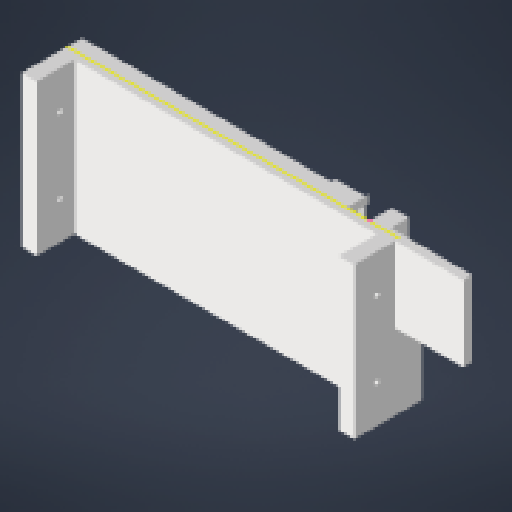
# Autodesk Inventor part: offloadbase
Saved by Autodesk Inventor 2027 (Build 310192000, 192)
## iProperties
Created: 2026-07-10
Part Number: offloadbase
Material: Generic
Document SubType Name: Modeling
Designer: uchiha
Density: 1 g/cm^3
Appearance: Default
Mass: 216.728 g
Surface Area: 672.485 cm^2
Volume: 216.728 cm^3
Author: uchiha
Autodesk Inventor part; units mm, degrees
sketch "Sketch1" plane through (0, 0, 0) normal (0, 0, 1) x (1, 0, 0)
  line L0 (-110, 50) -> (110, 50)
  line L1 (110, 50) -> (110, -50)
  line L2 (110, -50) -> (-110, -50)
  line L3 (-110, -50) -> (-110, 50)
  line L4 (-110, 50) -> (110, -50) construction
  line L5 (110, 50) -> (-110, -50) construction
  line L6 (110, 50) -> (100, 50)
  line L7 (100, 50) -> (100, -50)
  line L8 (100, -50) -> (110, -50)
  line L9 (110, -50) -> (110, 50)
  line L10 (-110, 50) -> (-100, 50)
  line L11 (-100, 50) -> (-100, -50)
  line L12 (-100, -50) -> (-110, -50)
  line L13 (-110, -50) -> (-110, 50)
  point P0 (0, 0)
  dimension "d0" = 220
  dimension "d1" = 100
  dimension "d2" = 10
  dimension "d3" = 10
  constraints: 28 end point, 6 parallel, 3 horizontal, 3 perpendicular, 2 midpoint, 2 point on line
  measures "d0" distance of L1.end L2.end
  measures "d1" distance of L0.end L1.end
  measures "d2" distance of L8.end L7.end
  measures "d3" distance of L11.end L12.end
extrude "Extrusion1" add sketch "Sketch1" along normal blind 5 contours L0 L7 L2 L11
extrude "Extrusion2" add sketch "Sketch1" along normal blind 30 contours L0 L11 L2 L3 | L0 L1 L2 L7
sketch "Sketch2" plane through (110, -50, 0) normal (1, 0, 0) x (0, 0, -1)
  circle A0 centre (-15, 75) radius 1.5
  circle A1 centre (-15, 25) radius 1.5
  line L0 (0, 100) -> (-30, 100) projected
  line L1 (0, 0) -> (-30, 0) projected
  point P0 (0, 50)
  point P1 (-15, 100)
  point P2 (-15, 0)
  dimension "d8" = 3
  dimension "d9" = 3
  dimension "d10" = 25
  dimension "d11" = 25
  constraints: 2 centre point, 2 midpoint
  measures "d8" diameter of A0
  measures "d9" diameter of A1
  measures "d10" distance of point (-15, 100) A0.centre
  measures "d11" distance of point (-15, 0) A1.centre
extrude "Extrusion3" cut sketch "Sketch2" against normal blind 300
ref_plane "Work Plane1" through (0, 0, 2.5) normal (0, 0, -1) x (-1, 0, 0)
sketch "Sketch5" plane through (-100, -50, 5) normal (0, -1, 0) x (1, 0, 0)
  point P0 (100, -5)
sketch "Sketch6" plane through (0, 0, 0) normal (0, 0, -1) x (-1, 0, 0)
  line L0 (-110, 50) -> (110, 50) projected
  line L1 (-90, 50) -> (-75, 50)
  point P0 (0, 0)
  constraints: 2 end point, 1 horizontal
sketch "Sketch7" plane through (-100, -50, 5) normal (0, -1, 0) x (1, 0, 0)
  point P0 (100, -5)
sketch "Sketch10" plane through (0, 0, 0) normal (0, 0, -1) x (-1, 0, 0)
  point P0 (0, 0)
sketch "Sketch11" plane through (-100, -50, 5) normal (0, -1, 0) x (1, 0, 0)
  point P0 (100, -5)
sketch "Sketch12" plane through (-100, -50, 5) normal (0, -1, 0) x (1, 0, 0)
  point P0 (100, -5)
sketch "Sketch13" plane through (-100, -50, 5) normal (0, -1, 0) x (1, 0, 0)
  point P0 (100, -5)
sketch "Sketch14" plane through (-100, -50, 5) normal (0, -1, 0) x (1, 0, 0)
  point P0 (100, -5)
ref_plane "Work Plane3" through (-100, -40, 5) normal (0, -1, 0) x (1, 0, 0)
sketch "Sketch16" plane through (0, 0, 0) normal (0, 0, -1) x (-1, 0, 0)
  point P0 (0, 0)
sketch "Sketch18" plane through (-100, -50, 5) normal (0, -1, 0) x (1, 0, 0)
  point P0 (100, -5)
sketch "Sketch20" plane through (0, 0, 0) normal (0, 0, -1) x (-1, 0, 0)
  line L0 (-110, 50) -> (110, 50) projected
  line L1 (100, -50) -> (-100, -50) projected
  line L2 (-110, 50) -> (-90, 50)
  line L3 (-90, 50) -> (-90, -50)
  line L4 (-90, -50) -> (-110, -50)
  line L5 (-110, -50) -> (-110, 50)
  line L6 (-100, 50) -> (100, 50) projected
  line L7 (-74.75, 50) -> (-54.75, 50)
  line L8 (-54.75, 50) -> (-54.75, -50)
  line L9 (-54.75, -50) -> (-74.75, -50)
  line L10 (-74.75, -50) -> (-74.75, 50)
  point P0 (0, 0)
  point P1 (-74.75, 50)
  point P2 (-74.75, -50)
  dimension "d46" = 20
  dimension "d47" = 20
  dimension "d48" = 15.25
  constraints: 16 end point, 4 parallel, 3 point on line, 2 horizontal, 2 perpendicular
  measures "d46" distance of L3.end L4.end
  measures "d47" distance of L8.end L9.end
  measures "d48" distance between parallel lines of L10 L3
extrude "Extrusion10" add sketch "Sketch20" along normal blind 15 contours L0 L3 L1 L4 L5 | L0 L8 L1 L10
ref_plane "Work Plane5" through (-100, -50, 5) normal (0, -1, 0) x (1, 0, 0)
sketch "Sketch22" plane through (-100, -50, 5) normal (0, -1, 0) x (1, 0, 0)
  line L0 (174.75, -5) -> (190, -5) projected
  line L1 (182.375, -5) -> (182.375, -19.781)
  arc A0 (174.1976, -13.8453) -> (174.1552, -16.1739) centre (172.7726, -14.984) ccw
  arc A1 (174.184, -13.8286) -> (174.1552, -16.1739) centre (172.7726, -14.984) ccw
  arc A2 (174.184, -13.8286) -> (174.5946, -13.637) centre (174.3446, -13.637) ccw
  line L2 (174.5946, -13.637) -> (174.5946, -4.5959)
  line L3 (174.5946, -4.5959) -> (190.095, -4.5959)
  line L4 (190.095, -4.5959) -> (190.095, -13.6504)
  arc A3 (190.095, -13.6504) -> (190.5052, -13.8286) centre (190.3446, -13.637) ccw
  arc A4 (190.5341, -16.1739) -> (190.5052, -13.8286) centre (191.9167, -14.984) ccw
  arc A5 (190.5341, -16.1739) -> (190.0946, -16.337) centre (190.3446, -16.337) ccw
  line L5 (190.0946, -16.337) -> (190.0946, -19.8904)
  line L6 (190.0946, -19.8904) -> (174.5946, -19.8904)
  line L7 (174.5946, -19.8904) -> (174.5946, -16.337)
  arc A6 (174.5946, -16.337) -> (174.1552, -16.1739) centre (174.3446, -16.337) ccw
  line L8 (174.75, -5) -> (174.75, -20) projected
  circle A7 centre (182.375, -12.3905) radius 0.9755 construction
  line L9 (190, -5) -> (190, -20) projected
  line L10 (154.75, -5) -> (154.75, -20) projected
  line L11 (174.75, -20) -> (154.75, -20)
  line L12 (154.75, -20) -> (154.75, -18)
  line L13 (154.75, -18) -> (174.75, -18)
  line L14 (174.75, -18) -> (174.75, -20)
  point P0 (100, -5)
  point P1 (182.7765, -10.9918)
  point P2 (174.184, -13.8286)
  point P3 (174.75, -19.8904)
  point P4 (190, -19.8904)
  point P5 (174.5946, -18)
  dimension "d74" = 2
  constraints: 22 end point, 14 point on circle, 8 centre point, 2 midpoint, 2 parallel, 1 horizontal, 1 perpendicular, 1 point on line, 1 vertical
  measures "d74" distance of L11.end L12.end
extrude "Extrusion13" cut sketch "Sketch22" against normal blind 95 contours L8 L13 L7 A6 A0 A2 L2 L3 L4 A3 A4 A5 L5 L6 L9 L0 | L8 L6 L7 L13
sketch "Sketch23" plane through (0, 0, 0) normal (0, 0, -1) x (-1, 0, 0)
  line L0 (110, -50) -> (-54.75, -50) projected
  line L1 (-54.75, 50) -> (-54.75, -50) projected
  line L2 (110, -50) -> (-54.75, -50)
  line L3 (-54.75, -50) -> (-54.75, 50)
  line L4 (-54.75, 50) -> (110, 50)
  line L5 (110, 50) -> (110, -50)
  point P0 (0, 0)
  constraints: 8 end point, 2 parallel, 1 horizontal, 1 perpendicular
extrude "Extrusion14" add sketch "Sketch23" along normal blind 10
extrude "Extrusion15" cut sketch "Sketch22" against normal blind 100 contours L8 L11 L10 L13 L7 L6
sketch "Sketch24" plane through (110, -50, 30) normal (1, 0, 0) x (0, 0, -1)
  line L0 (45, 100) -> (0, 100) projected
  line L1 (45, 100) -> (33.2, 100)
  line L2 (33.2, 100) -> (33.2, 50)
  line L3 (33.2, 50) -> (45, 50)
  line L4 (45, 50) -> (45, 100)
  point P0 (30, 50)
  dimension "d77" = 11.8
  constraints: 8 end point, 2 parallel, 1 horizontal, 1 perpendicular
  measures "d77" distance of L3.end L2.end
extrude "Extrusion16" cut sketch "Sketch24" against normal blind 9
sketch "Sketch25" plane through (110, -50, 30) normal (1, 0, 0) x (0, 0, -1)
  line L0 (40, 100) -> (0, 100) projected
  line L1 (33.2, 100) -> (23.2, 100)
  line L2 (23.2, 100) -> (23.2, 50)
  line L3 (23.2, 50) -> (33.2, 50)
  line L4 (33.2, 50) -> (33.2, 100)
  line L5 (33.2, 50) -> (33.2, 100) projected
  point P0 (30, 50)
  dimension "d80" = 10
  constraints: 8 end point, 2 parallel, 1 collinear, 1 horizontal, 1 perpendicular, 1 point on line
  measures "d80" distance of L3.end L2.end
extrude "Extrusion17" add sketch "Sketch25" along normal blind 45
sketch "Sketch26" plane through (110, 0, 6.8) normal (0, 0, 1) x (1, 0, 0)
  line L0 (0, 0) -> (0, 50) projected
  line L1 (0, 0) -> (45, 0) projected
  line L2 (45, 50) -> (45, 0) projected
  line L3 (0, 50) -> (45, 50) projected
  point P0 (-110, 0)
extrude "Extrusion18" cut sketch "Sketch26" against normal blind 4
body "Solid1"
